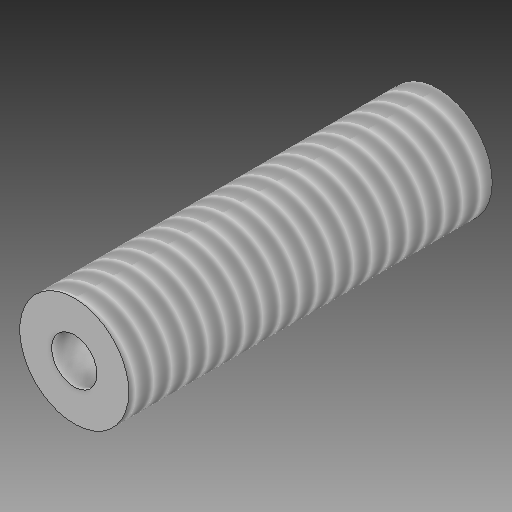
# Autodesk Inventor part: DüseGewinde
Saved by Autodesk Inventor 2021 (Build 250183000, 183)
## iProperties
Created: 2021-07-20
Part Number: DüseGewinde
Material: Generisch
Document SubType Name: Modeling
Designer: lukas
Density: 1 g/cm^3
Appearance: Vorgabe
Author: lukas
Autodesk Inventor part; units mm, degrees
ref_plane "YZ Plane" through (0, 0, 0) normal (1, 0, 0) x (0, 1, 0)
ref_plane "XZ Plane" through (0, 0, 0) normal (0, 1, 0) x (-1, 0, 0)
ref_plane "XY Plane" through (0, 0, 0) normal (0, 0, 1) x (1, 0, 0)
sketch "Skizze1" plane through (0, 0, 0) normal (0, 0, 1) x (1, 0, 0)
  line L0 (-4.2, 0) -> (4.2, 0) projected
  line L1 (0, -4.2) -> (0, 4.2) projected
  circle A0 centre (0, 0) radius 3
  circle A1 centre (0, 0) radius 1.25
  dimension "d0" = 6
  dimension "d1" = 2.5
  constraints: 2 centre point, 2 coincident
  measures "d0" diameter of A0
  measures "d1" diameter of A1
extrude "Extrusion1" add sketch "Skizze1" against normal blind 20 contours A1 L1 A0 L0 | L0 A0 L1 A1 | A1 L0 A0 L1 | L1 A0 L0 A1
thread "Gewinde1" size "M6x1" class "6g" standard "ANSI Metric M Profile" full length
